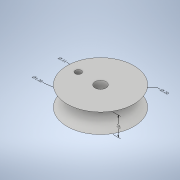
# Autodesk Inventor part: LittleBigWheel
Saved by Autodesk Inventor 2020 (Build 240168000, 168)
## iProperties
Created: 2019-12-13
Part Number: LittleBigWheel
Material: Generic
Document SubType Name: Modeling
Designer: AOFUser
Density: 1 g/cm^3
Appearance: Default
Author: AOFUser
Autodesk Inventor part; units mm, degrees
ref_plane "YZ Plane" through (0, 0, 0) normal (1, 0, 0) x (0, 1, 0)
ref_plane "XZ Plane" through (0, 0, 0) normal (0, 1, 0) x (-1, 0, 0)
ref_plane "XY Plane" through (0, 0, 0) normal (0, 0, 1) x (1, 0, 0)
sketch "Sketch1" plane through (0, 0, 0) normal (0, 1, 0) x (-1, 0, 0)
  circle A0 centre (0, 0) radius 15.24
  dimension "d0" = 30.48
  constraints: 1 centre point, 1 coincident
  measures "d0" diameter of A0
extrude "Extrusion1" add sketch "Sketch1" along normal blind 4.445
draft "FaceDraft1" angle 60 pull direction (0, 1, 0) faces at (-15.1906, 2.9633, -1.2263) fixed edges at (15.24, 0, 0)
sketch "Sketch2" plane through (0, 4.445, 0) normal (0, 1, 0) x (1, 0, 0)
  circle A0 centre (0, 0) radius 15.24
  constraints: 1 centre point, 1 coincident
extrude "Extrusion2" add sketch "Sketch2" along normal blind 4.445
draft "FaceDraft2" angle 60 pull direction (0, -1, 0) faces at (15.1906, 7.4083, 1.2263) fixed edges at (-15.24, 8.89, 0)
sketch "Sketch3" plane through (0, 8.89, 0) normal (0, 1, 0) x (1, 0, 0)
  circle A0 centre (0, 0) radius 15.24 projected
  line L0 (-15.24, 0) -> (0, 0)
  constraints: 2 end point, 1 horizontal, 1 horizontal alignment, 1 other
hole "Hole1" at (0, 8.89, 0) direction (0, -1, 0) diameter 5.08 end through all
sketch "Sketch4" plane through (0, 8.89, 0) normal (0, 1, 0) x (1, 0, 0)
  circle A0 centre (0, 0) radius 2.54 projected
  line L0 (-2.54, 0) -> (-10.16, 0)
  dimension "d14" = 7.62
  constraints: 2 end point, 1 horizontal, 1 horizontal alignment, 1 other
  measures "d14" distance of L0.start L0.end
hole "Hole2" at (-10.16, 8.89, 0) direction (0, -1, 0) diameter 2.794 end through all
body "Solid1"
